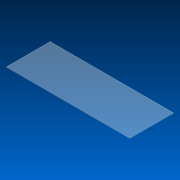
# Autodesk Inventor part: lead
Saved by Autodesk Inventor 2012 (Build 160160000, 160)
## iProperties
Created: 2012-07-04
Part Number: lead
Material: Default
Document SubType Name: Modeling
Designer: Hemant
Density: 1 g/cm^3
Author: Hemant
Autodesk Inventor part; units mm, degrees
ref_plane "YZ Plane" through (0, 0, 0) normal (1, 0, 0) x (0, 1, 0)
ref_plane "XZ Plane" through (0, 0, 0) normal (0, 1, 0) x (-1, 0, 0)
ref_plane "XY Plane" through (0, 0, 0) normal (0, 0, 1) x (1, 0, 0)
sketch "Sketch1" plane through (0, 0, 0) normal (0, 0, 1) x (1, 0, 0)
  line L0 (0, 0) -> (1219.2, 0)
  line L1 (1219.2, 0) -> (1219.2, 6.35)
  line L2 (1219.2, 6.35) -> (0, 6.35)
  line L3 (0, 6.35) -> (0, 0)
  dimension "d0" = 6.35
  dimension "d1" = 1219.2
  constraints: 8 end point, 2 parallel, 1 horizontal, 1 perpendicular
  measures "d0" distance between parallel lines of L2 L0
  measures "d1" distance between parallel lines of L1 L3
extrude "Extrusion1" add sketch "Sketch1" against normal blind 431.8
body "Solid1"
